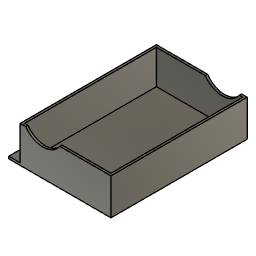
Water_holder (Autodesk Fusion 360 design; units mm, degrees)
Autodesk Fusion 360 part; units mm, degrees
sketch "Sketch1" plane through (0, 0, 0) normal (0, 0, 1) x (1, 0, 0)
  line L0 (0, 0) -> (90, 0)
  line L1 (90, 0) -> (90, 120)
  line L2 (90, 120) -> (0, 120)
  line L3 (0, 120) -> (0, 0)
  circle A0 centre (5, 35) radius 2
  circle A1 centre (5, 85) radius 2
  dimension "d1" = 90
  dimension "d2" = 120
  dimension "d4" = 4
  dimension "d9" = 35
  dimension "d10" = 5
  dimension "d43" = 0
  dimension "d44" = 50
  constraint horizontal L0
  constraint vertical L1
  constraint horizontal L2
  constraint vertical L3
  constraint coincident L0.start L3.end
  measures "d1" distance of L0.start L0.end
  measures "d2" distance of L0.start L2.end
  measures "d4" diameter of A0
  measures "d9" distance of L0 A0.centre
  measures "d10" distance of L3 A0.centre
extrude "Extrude1" add sketch "Sketch1" along normal blind 2
sketch "Sketch2" plane through (0, 0, 2) normal (0, 0, 1) x (-1, 0, 0)
  circle A0 centre (-5, -35) radius 2
  line L0 (0, -120) -> (0, 0)
  line L1 (0, 0) -> (-90, 0)
  line L2 (-90, 0) -> (-90, -120)
  line L3 (-90, -120) -> (0, -120)
  line L4 (-90, 0) -> (-10, 0)
  line L5 (-10, 0) -> (-10, -120)
  line L6 (-10, -120) -> (-90, -120)
  line L7 (-90, -120) -> (-90, 0)
  line L8 (-10, -120) -> (-90, -120)
  line L9 (-90, -120) -> (-90, -118)
  line L10 (-90, -118) -> (-10, -118)
  line L11 (-10, -118) -> (-10, -120)
  line L12 (-10, -120) -> (-12, -120)
  line L13 (-12, -120) -> (-12, 0)
  line L14 (-12, 0) -> (-10, 0)
  line L15 (-10, 0) -> (-10, -120)
  line L16 (-90, 0) -> (-10, 0)
  line L17 (-10, 0) -> (-10, -2)
  line L18 (-10, -2) -> (-90, -2)
  line L19 (-90, -2) -> (-90, 0)
  line L20 (-90, 0) -> (-88, 0)
  line L21 (-88, 0) -> (-88, -120)
  line L22 (-88, -120) -> (-90, -120)
  line L23 (-90, -120) -> (-90, 0)
  circle A1 centre (-5, -85) radius 2
  dimension "d13" = 2
  dimension "d14" = 2
  dimension "d15" = 120
  dimension "d16" = 2
  dimension "d17" = 2
  constraint horizontal L4
  constraint vertical L5
  constraint horizontal L6
  constraint vertical L7
  constraint coincident L3 L5.end
  constraint coincident L1.end L2.start
  constraint horizontal L8
  constraint vertical L9
  constraint horizontal L10
  constraint vertical L11
  constraint horizontal L12
  constraint vertical L13
  constraint horizontal L14
  constraint vertical L15
  constraint horizontal L16
  constraint vertical L17
  constraint horizontal L18
  constraint vertical L19
  constraint horizontal L20
  constraint vertical L21
  constraint horizontal L22
  constraint vertical L23
  measures "d13" distance of L5.end L10.end
  measures "d14" distance of L5.end L12.end
  measures "d15" distance of L5.end L4.end
  measures "d16" distance of L1.end L18.end
  measures "d17" distance of L1.end L20.end
extrude "Extrude2" add sketch "Sketch2" along normal blind 30 contours L3 L5 L6 L8 L10 L11 L12 L13 L15 | L1 L4 L5 L13 L14 L15 L16 L17 L18 | L3 L6 L8 L10 L13 L21 | L5 L10 L13 L15 L18 | L1 L4 L13 L16 L18 L21 | L2 L3 L6 L7 L8 L9 L10 L21 L22 L23 | L1 L2 L4 L7 L16 L18 L19 L20 L21 L23 | L2 L7 L10 L18 L21 L23
sketch "Sketch3" plane through (0, 120, 0) normal (0, 1, 0) x (-1, 0, 0)
  line L0 (-90, 0) -> (0, 0)
  line L1 (0, 0) -> (0, 2)
  line L2 (0, 2) -> (-10, 2)
  line L3 (-10, 2) -> (-10, 32)
  line L4 (-10, 32) -> (-90, 32)
  line L5 (-90, 32) -> (-90, 0)
  circle A0 centre (-70, 42) radius 18
  line L6 (-88, 2) -> (-88, 32)
  dimension "d20" = 36
  dimension "d26" = 18
  dimension "d39" = 42
  measures "d20" diameter of A0
  measures "d26" distance of A0.centre L6
  measures "d39" distance of L0 A0.centre
sketch "Sketch4" plane through (0, 0, 0) normal (0, -1, 0) x (1, 0, 0)
  line L0 (0, 0) -> (90, 0)
  line L1 (90, 0) -> (90, 32)
  line L2 (90, 32) -> (10, 32)
  line L3 (10, 32) -> (10, 2)
  line L4 (10, 2) -> (0, 2)
  line L5 (0, 2) -> (0, 0)
  circle A0 centre (30, 42) radius 18
  line L6 (12, 2) -> (12, 32)
  dimension "d28" = 36
  dimension "d29" = 18
  dimension "d40" = 42
  measures "d28" diameter of A0
  measures "d29" distance of A0.centre L6
  measures "d40" distance of L0 A0.centre
hole "Hole1" at (30, 0, 42) direction (0, 1, 0) diameter 36 depth 4 tip angle 180
hole "Hole2" at (70, 120, 42) direction (0, -1, 0) diameter 36 depth 20 tip angle 118
